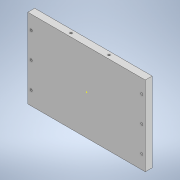
# Autodesk Inventor part: back
Saved by Autodesk Inventor 2022.2 (Build 262287030, 287C)
## iProperties
Created: 2022-01-28
Part Number: back
Material: Generic
Document SubType Name: Modeling
Designer: Tapendra
Density: 1 g/cm^3
Appearance: Default
Author: Tapendra
Autodesk Inventor part; units mm, degrees
ref_plane "YZ Plane" through (0, 0, 0) normal (1, 0, 0) x (0, 1, 0)
ref_plane "XZ Plane" through (0, 0, 0) normal (0, 1, 0) x (-1, 0, 0)
ref_plane "XY Plane" through (0, 0, 0) normal (0, 0, 1) x (1, 0, 0)
sketch "Sketch1" plane through (0, 0, 0) normal (0, 0, 1) x (1, 0, 0)
  line L0 (-85, 57.5) -> (85, 57.5)
  line L1 (85, 57.5) -> (85, -57.5)
  line L2 (85, -57.5) -> (-85, -57.5)
  line L3 (-85, -57.5) -> (-85, 57.5)
  line L4 (-85, 57.5) -> (85, -57.5) construction
  line L5 (85, 57.5) -> (-85, -57.5) construction
  point P0 (0, 0)
  dimension "d0" = 170
  dimension "d1" = 115
  constraints: 12 end point, 2 midpoint, 2 parallel, 1 horizontal, 1 perpendicular
  measures "d0" distance of L0.start L0.end
  measures "d1" distance of L0.end L1.end
extrude "Extrusion1" add sketch "Sketch1" along normal mid plane 10
sketch "Sketch2" plane through (0, 0, 5) normal (0, 0, 1) x (1, 0, 0)
  line L0 (-85, 57.5) -> (-85, -57.5) projected
  line L1 (-85, -57.5) -> (85, -57.5) projected
  point P0 (0, 0)
  point P1 (-80, -37.5)
  point P2 (80, -37.5)
  point P3 (-80, 0)
  point P4 (80, 0)
  point P5 (80, 37.5)
  point P6 (-80, 37.5)
  dimension "d58" = 10
  dimension "d4" = 5
  dimension "d5" = 20
  dimension "d11" = 160
  dimension "d55" = 37.5
  dimension "d62" = 37.5
  constraints: 2 vertical, 4 other
  measures "d4" distance from line of L0 point (-80, -37.5)
  measures "d5" distance from line of L1 point (-80, -37.5)
  measures "d11" distance of point (-80, -37.5) point (80, -37.5)
  measures "d55" distance of point (-80, -37.5) point (-80, 0)
  measures "d62" distance of point (80, -37.5) point (80, 0)
hole "Hole1" at (-80, -37.5, 5) at (-80, 0, 5) at (80, 0, 5) at (80, -37.5, 5) at (-80, 37.5, 5) at (80, 37.5, 5) direction (0, 0, -1) diameter 3.175 depth 5
sketch "Sketch3" plane through (-85, -57.5, 5) normal (0, -1, 0) x (1, 0, 0)
  line L0 (0, 0) -> (0, -10) projected
  line L1 (0, 0) -> (170, 0) projected
  point P0 (85, -5)
  point P1 (10, -5)
  point P2 (60, -5)
  point P3 (110, -5)
  point P4 (160, -5)
  dimension "d55" = 37.5
  dimension "d58" = 10
  dimension "d21" = 10
  dimension "d22" = 5
  dimension "d25" = 50
  constraints: 1 horizontal, 3 other
  measures "d21" distance from line of L0 point (10, -5)
  measures "d22" distance from line of L1 point (10, -5)
  measures "d25" distance of point (10, -5) point (60, -5)
hole "Hole2" at (-75, -57.5, 0) at (-25, -57.5, 0) at (25, -57.5, 0) at (75, -57.5, 0) direction (0, 1, 0) diameter 3.175 depth 5
sketch "Sketch4" plane through (-85, 57.5, 5) normal (0, 1, 0) x (1, 0, 0)
  line L0 (0, 10) -> (0, 0) projected
  line L1 (170, 0) -> (0, 0) projected
  line L2 (0, 10) -> (170, 10) projected
  point P0 (85, 5)
  point P1 (112.5, 5)
  point P2 (57.5, 5)
  dimension "d67" = 5
  dimension "d69" = 27.5
  dimension "d72" = 55
  constraints: 1 horizontal, 1 other
  measures "d67" distance from line of L2 point (112.5, 5)
  measures "d69" distance of point (85, 5) point (112.5, 5)
  measures "d72" distance of point (112.5, 5) point (57.5, 5)
hole "Hole3" at (27.5, 57.5, 0) at (-27.5, 57.5, 0) direction (0, -1, 0) diameter 3.175 depth 5
sketch "Sketch5" plane through (0, 0, 5) normal (0, 0, 1) x (1, 0, 0)
  point P0 (0, 0)
body "Solid1"
